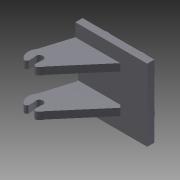
# Autodesk Inventor part: 2415
Saved by Autodesk Inventor 2011 SP1 (Build 150282100, 282)
## iProperties
Company: Allseas Engineering BV
Created: 2011-09-28
Part Number: 2415
Cost Center: 0 kg
Material: Steel
Document SubType Name: Modeling
Designer: PMe
Authority: 0 mm^3
Stock Number: =<Filenr>_<Document number>
Density: 7.85 g/cm^3
Act. Code: DW000
SaveDate: 2011-07-28
SaveTime: 18:32
FileName: Standard
TotalMass: 0 kg
TotalVolume: 0 mm^3
Subject: =<Title><TITLE 1_2> <TITLE 2_2>
Author: PMe
Autodesk Inventor part; units mm, degrees
ref_plane "YZ Plane" through (0, 0, 0) normal (1, 0, 0) x (0, 1, 0)
sketch "Sketch1" plane through (0, 0, 0) normal (0, 0, 1) x (1, 0, 0)
  line L0 (-8, 1.6) -> (8, 1.6)
  line L1 (8, 1.6) -> (8, 0)
  line L2 (8, 0) -> (-8, 0)
  line L3 (-8, 0) -> (-8, 1.6)
  arc A0 (-7.3, -8.3873) -> (-8.7, -8.3873) centre (-8, -8) ccw
  line L4 (-8.7, -8.3873) -> (-8.7, -10.4)
  line L5 (-7.3, -8.3873) -> (-7.3, -10.4)
  line L6 (-8, 0) -> (-10, -6.5)
  line L7 (-5.7087, -9) -> (2, 0)
  arc A1 (-7.3, -10.4) -> (-5.7087, -9) centre (-8, -8) ccw
  arc A2 (-10, -6.5) -> (-8.7, -10.4) centre (-8, -8) ccw
  point P0 (0, 0)
  point P1 (0, 0)
  dimension "d0" = 1.6
  dimension "d1" = 16
  dimension "d3" = 9.6
  dimension "d4" = 1.6
  dimension "d6" = 1.4
  dimension "d7" = 0.7
  dimension "d8" = 1
  dimension "d9" = 1.5
  dimension "d10" = 2.5
  dimension "d11" = 2.5
  dimension "d12" = 10
  constraints: 16 end point, 6 point on circle, 3 centre point, 2 coincident, 2 parallel, 2 vertical, 1 horizontal, 1 midpoint, 1 perpendicular, 1 point on line, 1 vertical alignment
  measures "d0" distance of L0.end L1.end
  measures "d1" distance of L0.start L0.end
  measures "d3" distance from line of L0 A0.centre
  measures "d4" diameter of A0
  measures "d6" distance between parallel lines of L5 L4
  measures "d7" distance from line of A0.centre L4
  measures "d8" vertical distance of A0.centre L7.start
  measures "d9" vertical distance of L6.end A0.centre
  measures "d10" radius of A1
  measures "d11" radius of A2
  measures "d12" distance of L2.end L7.end
extrude "Extrusion1" add sketch "Sketch1" along normal mid plane 16 contours L0 L1 L2 L3
ref_plane "Work Plane1" through (0, 0, -3.5) normal (0, 0, 1) x (1, 0, 0)
ref_plane "Work Plane2" through (0, 0, 3.5) normal (0, 0, 1) x (1, 0, 0)
sketch "Sketch2" plane through (0, 0, 3.5) normal (0, 0, 1) x (1, 0, 0)
  line L0 (-8, 0) -> (-10, -6.5) projected
  arc A0 (-10, -6.5) -> (-8.7, -10.4) centre (-8, -8) ccw projected
  line L1 (-8.7, -8.3873) -> (-8.7, -10.4) projected
  arc A1 (-7.3, -8.3873) -> (-8.7, -8.3873) centre (-8, -8) ccw projected
  line L2 (-7.3, -8.3873) -> (-7.3, -10.4) projected
  arc A2 (-7.3, -10.4) -> (-5.7087, -9) centre (-8, -8) ccw projected
  line L3 (-5.7087, -9) -> (2, 0) projected
  line L4 (8, 0) -> (-8, 0) projected
  point P0 (0, 0)
extrude "Extrusion2" add sketch "Sketch2" along normal blind 1.6
sketch "Sketch3" plane through (0, 0, -3.5) normal (0, 0, 1) x (1, 0, 0)
  line L0 (-8, 0) -> (-10, -6.5) projected
  arc A0 (-10, -6.5) -> (-8.7, -10.4) centre (-8, -8) ccw projected
  line L1 (-8.7, -8.3873) -> (-8.7, -10.4) projected
  arc A1 (-7.3, -8.3873) -> (-8.7, -8.3873) centre (-8, -8) ccw projected
  line L2 (-7.3, -8.3873) -> (-7.3, -10.4) projected
  arc A2 (-7.3, -10.4) -> (-5.7087, -9) centre (-8, -8) ccw projected
  line L3 (-5.7087, -9) -> (2, 0) projected
  line L4 (8, 0) -> (-8, 0) projected
  point P0 (0, 0)
extrude "Extrusion3" add sketch "Sketch3" against normal blind 1.6
fillet "Fillet1" radius 0.5 4 edges at (-8.7, -10.4, 4.3) (-7.3, -10.4, 4.3) (-7.3, -10.4, -4.3) (-8.7, -10.4, -4.3)
sketch "Sketch4" plane through (-8, 1.6, 8) normal (0, 1, 0) x (1, 0, 0)
  line L0 (16, 16) -> (0, 16) projected
  line L1 (0, 0) -> (0, 16) projected
  circle A0 centre (4, 12) radius 2.5
  circle A1 centre (12, 12) radius 2.5
  circle A2 centre (12, 4) radius 2.5
  circle A3 centre (4, 4) radius 2.5
  circle A4 centre (4, 12) radius 1.5
  circle A5 centre (12, 12) radius 1.5
  circle A6 centre (12, 4) radius 1.5
  circle A7 centre (4, 4) radius 1.5
  point P0 (8, 8)
  dimension "d22" = 8
  dimension "d23" = 8
  dimension "d24" = 4
  dimension "d25" = 4
  dimension "d26" = 5
  dimension "d27" = 3
  constraints: 8 centre point, 6 equal radius, 4 coincident, 2 horizontal alignment, 2 vertical alignment
  measures "d22" distance of A0.centre A3.centre
  measures "d23" distance of A1.centre A0.centre
  measures "d24" distance from line of L0 A0.centre
  measures "d25" distance from line of L1 A0.centre
  measures "d26" diameter of A0
  measures "d27" diameter of A4
extrude "Extrusion4" add sketch "Sketch4" along normal blind 1.6
sketch "Sketch5" plane through (-8, 0, -8) normal (0, -1, 0) x (1, 0, 0)
  line L0 (0, 11.5) -> (10, 11.5)
  line L1 (10, 11.5) -> (10, 4.5)
  line L2 (10, 4.5) -> (0, 4.5)
  line L3 (0, 4.5) -> (0, 11.5)
  point P0 (8, 8)
  constraints: 8 end point, 2 parallel, 1 horizontal, 1 perpendicular
extrude "Extrusion5" cut sketch "Sketch5" against normal blind 0.6
equation "\"d7\" = 0.5 * d6"
body "Solid1"
